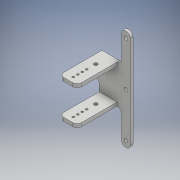
# Autodesk Inventor part: czesc_do_obudowy
Saved by Autodesk Inventor 2017 (Build 210142000, 142)
## iProperties
Created: 2019-10-29
Part Number: czesc_do_obudowy
Material: Ogólny
Document SubType Name: Modeling
Designer: patry
Density: 1 g/cm^3
Appearance: Domyślna
Author: patry
Autodesk Inventor part; units mm, degrees
ref_plane "YZ Plane" through (0, 0, 0) normal (1, 0, 0) x (0, 1, 0)
ref_plane "XZ Plane" through (0, 0, 0) normal (0, 1, 0) x (-1, 0, 0)
ref_plane "XY Plane" through (0, 0, 0) normal (0, 0, 1) x (1, 0, 0)
sketch "Szkic1" plane through (0, 0, 0) normal (0, 1, 0) x (-1, 0, 0)
  line L0 (9, 129.5) -> (-1, 129.5)
  line L1 (-1, 129.5) -> (-1, 15.5)
  line L2 (-1, 15.5) -> (9, 15.5)
  line L3 (9, 15.5) -> (9, 129.5)
  circle A0 centre (4, 22.5) radius 1.95
  circle A1 centre (4, 122.5) radius 1.95
  line L4 (48, 148) -> (48, 0)
  line L5 (9, 77.5) -> (48, 77.5)
  line L6 (48, 77.5) -> (48, 67.5)
  line L7 (48, 67.5) -> (9, 67.5)
  line L8 (9, 67.5) -> (9, 77.5)
  circle A2 centre (44, 72.5) radius 1.95
  line L9 (34, 94) -> (9, 94)
  line L10 (9, 94) -> (9, 51)
  line L11 (9, 51) -> (34, 51)
  line L12 (34, 51) -> (34, 94)
  circle A3 centre (4, 72.5) radius 1.95
  line L13 (34, 90) -> (9, 90) construction
  line L14 (9, 90) -> (9, 55) construction
  line L15 (9, 55) -> (34, 55) construction
  line L16 (34, 55) -> (34, 90) construction
  line L17 (34, 94) -> (14, 94)
  line L18 (14, 94) -> (14, 90)
  line L19 (14, 90) -> (34, 90)
  line L20 (34, 90) -> (34, 94)
  line L21 (14, 51) -> (34, 51)
  line L22 (34, 51) -> (34, 55)
  line L23 (34, 55) -> (14, 55)
  line L24 (14, 55) -> (14, 51)
  circle A4 centre (24, 47.5) radius 1.95
  circle A5 centre (24, 97.5) radius 1.95
  point P0 (0, 0)
  point P1 (12.3183, 7)
  dimension "d0" = 7
  dimension "d1" = 7
  dimension "d2" = 5
  dimension "d3" = 5
  dimension "d4" = 5
  dimension "d5" = 5
  dimension "d6" = 43
  dimension "d7" = 16.5
  dimension "d8" = 25
  dimension "d9" = 35
  dimension "d10" = 12.5
  dimension "d11" = 10
  constraints: 50 end point, 12 parallel, 8 point on line, 6 centre point, 6 horizontal, 6 perpendicular
  measures "d0" distance from line of L0 A1.centre
  measures "d1" distance from line of L2 A0.centre
  measures "d2" distance from line of L1 A0.centre
  measures "d3" distance from line of L3 A0.centre
  measures "d4" distance from line of L7 A2.centre
  measures "d5" distance from line of L5 A2.centre
  measures "d6" distance of L10.end L9.end
  measures "d7" distance between parallel lines of L7 L11
  measures "d8" distance between parallel lines of L3 L12
  measures "d9" distance of L14.end L13.end
  measures "d10" distance between parallel lines of L7 L15
  measures "d11" distance from line of A4.centre L24
extrude "Wyciągnięcie proste1" add sketch "Szkic1" along normal blind 3 contours L3 L2 L1 L0 | L9 L18 L19 L12 L5 L3 | L5 L12 L7 L3 | L9 L12 L19 L18 | L7 L12 L23 L24 L11 L3 | L5 L4 L7 L12 | L24 L23 L12 L11
extrude "Wyciągnięcie proste2" add sketch "Szkic1" against normal blind 45 contours L9 L12 L19 L18 | L24 L23 L12 L11
fillet "Zaokrąglenie1" radius 5 14 edges at (-34, 1.5, 67.5) (-34, 1.5, 77.5) (-48, 1.5, 77.5) (-48, 1.5, 67.5) (-9, 1.5, 51) (-9, 1.5, 15.5) (1, 1.5, 15.5) (-9, 1.5, 94) (-9, 1.5, 129.5) (1, 1.5, 129.5) (-34, -45, 92) (-34, -45, 53) (-14, -45, 53) (-14, -45, 92)
sketch "Szkic2" plane through (-14, 3, 51) normal (0, 0, -1) x (-1, 0, 0)
  arc A0 (0, -43) -> (5, -48) centre (5, -43) ccw projected
  line L0 (15, -48) -> (5, -48) projected
  arc A1 (15, -48) -> (20, -43) centre (15, -43) ccw projected
  line L1 (20, -43) -> (20, 0) projected
  line L2 (0, 0) -> (20, 0) projected
  line L3 (0, -3) -> (0, 0) projected
  line L4 (0, -3) -> (0, -43) projected
  line L5 (-5, -3) -> (20, -3) projected
  point P0 (-14, -3)
  point P1 (10, -17)
  point P2 (10, -27.25)
  point P3 (10, -32.25)
  point P4 (10, -37.25)
  point P5 (10, -42.25)
  dimension "d17" = 14
  dimension "d18" = 10
  dimension "d19" = 10.25
  dimension "d20" = 5
  dimension "d21" = 5
  dimension "d22" = 5
  constraints: 4 vertical alignment
  measures "d17" distance from line of point (10, -17) L5
  measures "d18" distance from line of L4 point (10, -17)
  measures "d19" distance of point (10, -17) point (10, -27.25)
  measures "d20" distance of point (10, -27.25) point (10, -32.25)
  measures "d21" distance of point (10, -32.25) point (10, -37.25)
  measures "d22" distance of point (10, -37.25) point (10, -42.25)
hole "Otwór1" at (-24, -24.25, 51) at (-24, -29.25, 51) at (-24, -34.25, 51) at (-24, -39.25, 51) direction (0, 0, 1) diameter 2.4 end through all clearance for "Śruba ze łbem płaskim obrobiona" size "M2" standard "ANSI Profil metryczny M"
hole "Otwór2" at (-24, -14, 51) direction (0, 0, 1) diameter 3.9 end through all clearance for "Śruba ze łbem płaskim obrobiona" size "M3.5" standard "ANSI Profil metryczny M"
equation "\"d3\" = d2"
equation "\"d5\" = d4"
